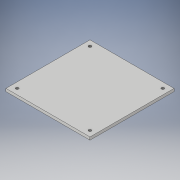
# Autodesk Inventor part: Grundplatte
Saved by Autodesk Inventor 2019.5 (Build 235369000, 369)
## iProperties
Created: 2021-09-30
Part Number: Grundplatte
Material: Generisch
Document SubType Name: Modeling
Designer: mritt
Density: 1 g/cm^3
Appearance: Vorgabe
Author: mritt
Autodesk Inventor part; units mm, degrees
ref_plane "YZ Plane" through (0, 0, 0) normal (1, 0, 0) x (0, 1, 0)
ref_plane "XZ Plane" through (0, 0, 0) normal (0, 1, 0) x (-1, 0, 0)
ref_plane "XY Plane" through (0, 0, 0) normal (0, 0, 1) x (1, 0, 0)
sketch "Skizze1" plane through (0, 0, 0) normal (0, 1, 0) x (-1, 0, 0)
  line L0 (144.9597, 31.6532) -> (-5.0403, 31.6532)
  line L1 (-5.0403, 31.6532) -> (-5.0403, -118.3468)
  line L2 (-5.0403, -118.3468) -> (144.9597, -118.3468)
  line L3 (144.9597, -118.3468) -> (144.9597, 31.6532)
  line L4 (144.9597, 31.6532) -> (-5.0403, -118.3468) construction
  line L5 (-5.0403, 31.6532) -> (144.9597, -118.3468) construction
  point P0 (0, 0)
  point P1 (69.9597, -43.3468)
  dimension "d0" = 150
  dimension "d1" = 150
  constraints: 12 end point, 2 midpoint, 2 parallel, 1 horizontal, 1 perpendicular
  measures "d0" distance of L0.end L1.end
  measures "d1" distance of L1.end L2.end
extrude "Extrusion1" add sketch "Skizze1" along normal blind 5
sketch "Skizze2" plane through (0, 5, 0) normal (0, 1, 0) x (1, 0, 0)
  circle A0 centre (-134.9597, -21.6532) radius 2.5
  circle A1 centre (-134.9597, 108.3468) radius 2.5
  circle A2 centre (-4.9597, -21.6532) radius 2.5
  circle A3 centre (-4.9597, 108.3468) radius 2.5
  line L0 (-144.9597, 118.3468) -> (-144.9597, -31.6532) projected
  line L1 (-144.9597, -31.6532) -> (5.0403, -31.6532) projected
  line L2 (5.0403, 118.3468) -> (-144.9597, 118.3468) projected
  line L3 (5.0403, -31.6532) -> (5.0403, 118.3468) projected
  point P0 (0, 0)
  dimension "d4" = 5
  dimension "d5" = 5
  dimension "d6" = 5
  dimension "d7" = 5
  dimension "d8" = 10
  dimension "d9" = 10
  dimension "d15" = 10
  dimension "d16" = 10
  dimension "d17" = 10
  dimension "d18" = 10
  dimension "d19" = 10
  dimension "d20" = 10
  constraints: 4 centre point
  measures "d4" diameter of A0
  measures "d5" diameter of A1
  measures "d6" diameter of A2
  measures "d7" diameter of A3
  measures "d8" distance from line of A0.centre L0
  measures "d9" distance from line of A0.centre L1
  measures "d15" distance from line of A1.centre L0
  measures "d16" distance from line of A1.centre L2
  measures "d17" distance from line of A2.centre L1
  measures "d18" distance from line of A2.centre L3
  measures "d19" distance from line of A3.centre L2
  measures "d20" distance from line of A3.centre L3
hole "Bohrung1" at (-134.9597, 5, 21.6532) at (-134.9597, 5, -108.3468) at (-4.9597, 5, -108.3468) at (-4.9597, 5, 21.6532) direction (0, -1, 0) diameter 4.978 depth 19.05 tip angle 118 thread size "1/4-20 UNC" class "2B" standard "ANSI Unified Screw Threads"
